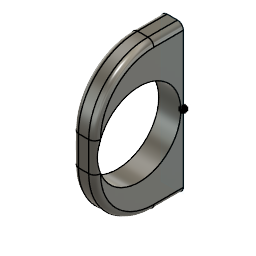
Atlas_Shelf_Truss_ST001 (Autodesk Fusion 360 archive; units mm, degrees)
design "Atlas_ShelfTab_ST001"
part number: 2026-07-26-16-47-24-662
Autodesk Fusion 360 part; units mm, degrees
sketch "Sketch1" plane through (0, 0, 0) normal (0, 0, 1) x (1, 0, 0)
  line L0 (0.9525, 6.35) -> (-0.9525, 6.35)
  line L1 (-0.9525, 6.35) -> (-0.9525, -6.35)
  line L2 (-0.9525, -6.35) -> (0.9525, -6.35)
  line L3 (0.9525, -6.35) -> (0.9525, 6.35)
  line L4 (0.9525, 6.35) -> (-0.9525, -6.35) construction
  line L5 (-0.9525, 6.35) -> (0.9525, -6.35) construction
  dimension "d7" = 1.905
  dimension "d8" = 12.7
  constraint horizontal L0
  constraint perpendicular L0 L1
  constraint parallel L0 L2
  constraint parallel L1 L3
  constraint coincident L4 origin
  constraint coincident L5 origin
  measures "d7" distance of L1.end L2.end
  measures "d8" distance of L0.end L1.end
extrude "Extrude1" add sketch "Sketch1" along normal blind 7.62
sketch "Sketch2" plane through (0.9525, 0, 0) normal (1, 0, 0) x (0, 0, -1)
  line L0 (0, -6.35) -> (0, 6.35)
  line L1 (0, 6.35) -> (-7.62, 6.35)
  line L2 (-7.62, 6.35) -> (-7.62, -6.35)
  line L3 (-7.62, -6.35) -> (0, -6.35)
  circle A0 centre (-3.7773, 0) radius 3.556
  dimension "d11" = 7.112
  measures "d11" diameter of A0
extrude "Extrude2" cut sketch "Sketch2" against normal blind 12.7 contours A0
sketch "Sketch3" plane through (0, 0, 0) normal (0, 0, -1) x (-1, 0, 0)
  line L0 (-0.9525, 6.35) -> (-0.9525, -6.35)
  line L1 (-0.9525, -6.35) -> (0.9525, -6.35)
  line L2 (0.9525, -6.35) -> (0.9525, 6.35)
  line L3 (0.9525, 6.35) -> (-0.9525, 6.35)
  point P0 (-0.9525, 0)
  constraint midpoint L0 P0
fillet "Fillet1" radius 5.08 2 edges at (0, 6.35, 7.62) (0, -6.35, 7.62)
fillet "Fillet2" radius 0.508 10 edges at (0.9525, -6.35, 1.27) (0.9525, -4.8621, 6.1321) (0.9525, 0, 7.62) (0.9525, 4.8621, 6.1321) (0.9525, 6.35, 1.27) (-0.9525, 6.35, 1.27) (-0.9525, 4.8621, 6.1321) (-0.9525, 0, 7.62) (-0.9525, -4.8621, 6.1321) (-0.9525, -6.35, 1.27)
equation "tabHeight = 0.3 in"
equation "tabWidth = 0.5 in"
equation "tabThickness = 0.075 in"
equation "pinSize = 0.25 in"
equation "pinHoleClearance = 0.03 in"
equation "pinHoleDiameter = pinSize + pinHoleClearance"
equation "d7 = tabThickness"
equation "d8 = tabWidth"
equation "d9 = tabHeight"
equation "d11 = pinHoleDiameter"
